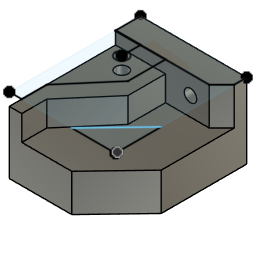
Robocon task1 image 1 v2 (Autodesk Fusion 360 design; units mm, degrees)
Autodesk Fusion 360 part; units mm, degrees
sketch "Sketch1" plane through (0, 0, 0) normal (0, 0, 1) x (1, 0, 0)
  line L0 (79.2263, -110) -> (-80.7737, -110)
  line L1 (-80.7737, -110) -> (-80.7737, 110)
  line L2 (-80.7737, 110) -> (79.2263, 110)
  line L3 (79.2263, 110) -> (79.2263, -110)
  line L4 (79.2263, -110) -> (-80.7737, 110) construction
  line L5 (-80.7737, -110) -> (79.2263, 110) construction
  point P0 (-0.7737, 0)
  dimension "d1" = 160
  dimension "d2" = 220
  constraint horizontal L0
  constraint perpendicular L0 L1
  constraint parallel L0 L2
  constraint parallel L1 L3
  constraint coincident L4 P0
  constraint coincident L5 P0
  measures "d1" distance of L1.end L2.end
  measures "d2" distance of L0.end L1.end
sketch "Sketch2" plane through (0, 0, 130) normal (0, 0, 1) x (-1, 0, 0)
  line L0 (-79.2263, -110) -> (80.7737, -110)
  line L1 (80.7737, -110) -> (80.7737, 110)
  line L2 (80.7737, 110) -> (-79.2263, 110)
  line L3 (-79.2263, 110) -> (-79.2263, -110)
  line L4 (-20, 110) -> (-79.2263, 29.9287)
  constraint coincident L2 L4.start
  constraint coincident L3 L4.end
sketch "Sketch3" plane through (0, 0, 0) normal (0, 0, 1) x (1, 0, 0)
  line L0 (85, -105) -> (-85, -105)
  line L1 (-85, -105) -> (-85, 105)
  line L2 (-85, 105) -> (85, 105)
  line L3 (85, 105) -> (85, -105)
  line L4 (85, -105) -> (-85, 105) construction
  line L5 (-85, -105) -> (85, 105) construction
  dimension "d7" = 170
  dimension "d8" = 210
  constraint horizontal L0
  constraint perpendicular L0 L1
  constraint parallel L0 L2
  constraint parallel L1 L3
  constraint coincident L4 origin
  constraint coincident L5 origin
  measures "d7" distance of L1.end L2.end
  measures "d8" distance of L0.end L1.end
extrude "Extrude3" add sketch "Sketch3" along normal blind 130
sketch "Sketch4" plane through (0, 0, 130) normal (0, 0, 1) x (-1, 0, 0)
  line L0 (-85, -105) -> (85, -105)
  line L1 (85, -105) -> (85, 105)
  line L2 (85, 105) -> (-85, 105)
  line L3 (-85, 105) -> (-85, -105)
  line L4 (-85, 105) -> (-15, 105)
  line L5 (-85, 101.8612) -> (-85, 31.8612)
  line L6 (-15, 105) -> (-85, 31.8612)
  line L7 (85, 105) -> (65, 105)
  line L8 (65, 105) -> (65, 65)
  line L9 (85, -105) -> (85, -65)
  line L10 (85, -65) -> (-65, -65)
  line L11 (-85, -105) -> (-85, -85)
  line L12 (-65, -65) -> (-85, -85)
  line L13 (85, -65) -> (5, -65)
  line L14 (5, -65) -> (5, -5)
  line L15 (5, -5) -> (65, 65)
  line L16 (85, -65) -> (45, -65)
  line L17 (45, -65) -> (45, -35)
  circle A0 centre (45, -35) radius 10
  dimension "d11" = 70
  dimension "d12" = 70
  dimension "d15" = 20
  dimension "d16" = 40
  dimension "d17" = 40
  dimension "d18" = 150
  dimension "d19" = 20
  dimension "d20" = 80
  dimension "d21" = 60
  dimension "d26" = 40
  dimension "d27" = 30
  dimension "d28" = 20
  constraint coincident L2.end L3.start
  constraint perpendicular L3 L4
  constraint coincident L3 L5.start
  constraint perpendicular L2 L5
  constraint coincident L1.end L2.start
  constraint perpendicular L1 L7
  constraint perpendicular L7 L8
  constraint coincident L0.end L1.start
  constraint perpendicular L0 L9
  constraint perpendicular L9 L10
  constraint coincident L0.start L3.end
  constraint perpendicular L0 L11
  constraint perpendicular L9 L13
  constraint perpendicular L10 L14
  constraint perpendicular L1 L16
  constraint perpendicular L10 L17
  constraint coincident L17.end A0.centre
  measures "d11" distance of L2.end L4.end
  measures "d12" distance of L5.start L5.end
  measures "d15" distance of L1.end L7.end
  measures "d16" distance of L7.end L8.end
  measures "d17" distance of L0.end L9.end
  measures "d18" distance of L9.end L10.end
  measures "d19" distance of L0.start L11.end
  measures "d20" distance of L9.end L13.end
  measures "d21" distance of L13.end L14.end
  measures "d26" distance of L9.end L16.end
  measures "d27" distance of L16.end L17.end
  measures "d28" diameter of A0
extrude "Extrude4" cut sketch "Sketch4" against normal blind 130 contours L2 L3 L4 L5 L6
extrude "Extrude5" cut sketch "Sketch4" against normal blind 60 contours L2 L3 L6 L8 L10 L12 L14 L15
extrude "Extrude6" cut sketch "Sketch4" against normal blind 20 contours L1 L2 L7 L8 L10 L13 L14 L15 L16 | A0
extrude "Extrude7" cut sketch "Sketch4" against normal blind 130 contours A0
sketch "Sketch5" plane through (0, 65, 0) normal (0, -1, 0) x (1, 0, 0)
  line L0 (65, 130) -> (-85, 130)
  line L1 (-85, 130) -> (-85, 110)
  line L2 (-85, 110) -> (-5, 110)
  line L3 (-5, 110) -> (-5, 70)
  line L4 (-5, 70) -> (65, 70)
  line L5 (65, 70) -> (65, 130)
  line L6 (65, 130) -> (35, 130)
  line L7 (35, 130) -> (35, 100)
  circle A0 centre (35, 100) radius 10
  dimension "d31" = 30
  dimension "d32" = 30
  dimension "d33" = 20
  constraint coincident L0.start L5.end
  constraint perpendicular L5 L6
  constraint perpendicular L6 L7
  constraint coincident L7.end A0.centre
  measures "d31" distance of L0.start L6.end
  measures "d32" distance of L6.end L7.end
  measures "d33" diameter of A0
extrude "Extrude8" cut sketch "Sketch5" against normal blind 40 contours A0
sketch "Sketch6" plane through (85, 0, 0) normal (1, 0, 0) x (0, 1, 0)
  line L0 (85, 130) -> (85, 70)
  line L1 (85, 70) -> (-31.8612, 70)
  line L2 (-31.8612, 70) -> (-31.8612, 0)
  line L3 (-31.8612, 0) -> (105, 0)
  line L4 (105, 0) -> (105, 130)
  line L5 (105, 130) -> (85, 130)
  line L6 (105, 0) -> (105, 10)
  line L7 (105, 10) -> (-105.2237, 10)
  dimension "d36" = 10
  constraint coincident L3.end L4.start
  constraint perpendicular L3 L6
  constraint perpendicular L2 L7
  measures "d36" distance of L3.end L6.end
extrude "Extrude9" cut sketch "Sketch6" against normal blind 300 contours L2 L3 L4 L6 L7
sketch "Sketch7" plane through (60.2783, -57.6914, 0) normal (0.722439, -0.691435, 0) x (0.691435, 0.722439, 0)
  line L0 (35.7542, 70) -> (-65.4846, 70)
  line L1 (-65.4846, 70) -> (-65.4846, 0)
  line L2 (-65.4846, 0) -> (35.7542, 0)
  line L3 (35.7542, 0) -> (35.7542, 10)
  line L4 (35.7542, 10) -> (35.7542, 70)
  line L5 (-65.4846, 0) -> (-65.4846, 10)
  line L6 (-65.4846, 10) -> (35.7542, 10)
  dimension "d39" = 10
  constraint coincident L1.end L2.start
  constraint perpendicular L2 L5
  constraint coincident L3.end L4.start
  measures "d39" distance of L1.end L5.end
extrude "Extrude10" cut sketch "Sketch7" against normal blind 399 contours L1 L2 L3 L5 L6
sketch "Sketch8" plane through (0, -105, 0) normal (0, -1, 0) x (1, 0, 0)
  line L0 (-65, 110) -> (-85, 110)
  line L1 (-85, 110) -> (-85, 0)
  line L2 (-85, 0) -> (15, 0)
  line L3 (15, 0) -> (15, 10)
  line L4 (15, 10) -> (15, 70)
  line L5 (15, 70) -> (-65, 70)
  line L6 (-65, 70) -> (-65, 110)
  line L7 (15, 10) -> (-85, 10)
  constraint coincident L3.end L4.start
  constraint coincident L1 L7.end
  constraint perpendicular L1 L7
extrude "Extrude11" cut sketch "Sketch8" against normal blind 300 contours L1 L2 L3 L7
